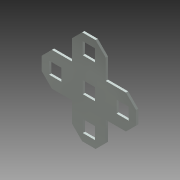
# Autodesk Inventor part: 276-1110
Saved by Autodesk Inventor 2013 (Build 170138000, 138)
## iProperties
Category: Structure
Company: Autodesk Inc.
Created: 2012-04-11
Part Number: 276-1110
Document SubType Name: Modeling
Designer: Autodesk Inc.
Density: 7.85 g/cm^3
Material: Steel
Catalog Web Link: http://www.vexrobotics.com/276-1110.html
Vendor: VEX
Mass: 3.81207 g
Surface Area: 13.3961 cm^2
Volume: 0.485614 cm^3
Author: Autodesk Inc.
Autodesk Inventor part; units mm, degrees
ref_plane "YZ Plane" through (0, 0, 0) normal (1, 0, 0) x (0, 1, 0)
ref_plane "XZ Plane" through (0, 0, 0) normal (0, 1, 0) x (-1, 0, 0)
ref_plane "XY Plane" through (0, 0, 0) normal (0, 0, 1) x (1, 0, 0)
sketch "Sketch1" plane through (0, 0, 0) normal (0, 0, 1) x (1, 0, 0)
  line L0 (20.9262, 6.7683) -> (20.9262, 1.6883)
  line L1 (-14.6338, 1.6883) -> (-14.6338, 6.7683)
  line L2 (0.6062, 22.0083) -> (5.6862, 22.0083)
  line L3 (5.6862, -13.5517) -> (0.6062, -13.5517)
  line L4 (-3.2038, -9.7417) -> (-3.2038, -2.1217)
  line L5 (-3.2038, 10.5783) -> (-3.2038, 18.1983)
  line L6 (-10.8238, 10.5783) -> (-3.2038, 10.5783)
  line L7 (9.4962, 10.5783) -> (17.1162, 10.5783)
  line L8 (17.1162, -2.1217) -> (9.4962, -2.1217)
  line L9 (-3.2038, -2.1217) -> (-10.8238, -2.1217)
  line L10 (9.4962, 18.1983) -> (9.4962, 10.5783)
  line L11 (9.4962, -2.1217) -> (9.4962, -9.7417)
  line L12 (-3.2038, 18.1983) -> (0.6062, 22.0083)
  line L13 (5.6862, 22.0083) -> (9.4962, 18.1983)
  line L14 (17.1162, 10.5783) -> (20.9262, 6.7683)
  line L15 (20.9262, 1.6883) -> (17.1162, -2.1217)
  line L16 (9.4962, -9.7417) -> (5.6862, -13.5517)
  line L17 (-3.2038, -9.7417) -> (0.6062, -13.5517)
  line L18 (-14.6338, 1.6883) -> (-10.8238, -2.1217)
  line L19 (-14.6338, 6.7683) -> (-10.8238, 10.5783)
  line L20 (0.8602, 19.2143) -> (5.4322, 19.2143)
  line L21 (5.4322, 19.2143) -> (5.4322, 14.6423)
  line L22 (5.4322, 14.6423) -> (0.8602, 14.6423)
  line L23 (0.8602, 14.6423) -> (0.8602, 19.2143)
  line L24 (-11.8398, 6.5143) -> (-7.2678, 6.5143)
  line L25 (-7.2678, 6.5143) -> (-7.2678, 1.9423)
  line L26 (-7.2678, 1.9423) -> (-11.8398, 1.9423)
  line L27 (-11.8398, 1.9423) -> (-11.8398, 6.5143)
  line L28 (0.8602, -6.1857) -> (5.4322, -6.1857)
  line L29 (5.4322, -6.1857) -> (5.4322, -10.7577)
  line L30 (5.4322, -10.7577) -> (0.8602, -10.7577)
  line L31 (0.8602, -10.7577) -> (0.8602, -6.1857)
  line L32 (13.5602, 6.5143) -> (18.1322, 6.5143)
  line L33 (18.1322, 6.5143) -> (18.1322, 1.9423)
  line L34 (18.1322, 1.9423) -> (13.5602, 1.9423)
  line L35 (13.5602, 1.9423) -> (13.5602, 6.5143)
  line L36 (0.8602, 6.5143) -> (5.4322, 6.5143)
  line L37 (5.4322, 6.5143) -> (5.4322, 1.9423)
  line L38 (5.4322, 1.9423) -> (0.8602, 1.9423)
  line L39 (0.8602, 1.9423) -> (0.8602, 6.5143)
  point P0 (-14.6338, 10.5783)
  point P1 (20.9262, -2.1217)
  point P2 (20.9262, 10.5783)
  point P3 (-14.6338, -2.1217)
  point P4 (-3.2038, 22.0083)
  point P5 (9.4962, -13.5517)
  point P6 (9.4962, 22.0083)
  point P7 (-3.2038, -13.5517)
  dimension "d0" = 35.56
  dimension "d1" = 35.56
  dimension "d2" = 12.7
  dimension "d3" = 12.7
  dimension "d4" = 12.7
  dimension "d5" = 12.7
  dimension "d6" = 11.43
  dimension "d7" = 11.43
  dimension "d8" = 11.43
  dimension "d9" = 11.43
  dimension "d10" = 3.81
  dimension "d11" = 3.81
  dimension "d12" = 3.81
  dimension "d13" = 3.81
  dimension "d14" = 3.81
  dimension "d15" = 3.81
  dimension "d16" = 3.81
  dimension "d17" = 3.81
  dimension "d18" = 3.81
  dimension "d19" = 3.81
  dimension "d20" = 3.81
  dimension "d21" = 3.81
  dimension "d22" = 3.81
  dimension "d23" = 3.81
  dimension "d24" = 3.81
  dimension "d25" = 3.81
  dimension "d26" = 4.572
  dimension "d27" = 4.572
  dimension "d28" = 4.572
  dimension "d29" = 4.572
  dimension "d30" = 4.572
  dimension "d31" = 4.572
  dimension "d32" = 4.572
  dimension "d33" = 4.572
  dimension "d34" = 4.572
  dimension "d35" = 4.572
  dimension "d36" = 2.794
  dimension "d37" = 2.794
  dimension "d38" = 2.794
  dimension "d39" = 2.794
  dimension "d40" = 4.064
  dimension "d41" = 4.064
  dimension "d42" = 11.43
  constraints: 80 end point, 20 parallel, 16 point on line, 9 perpendicular, 8 horizontal, 4 collinear
  measures "d0" distance between parallel lines of L0 L1
  measures "d1" distance between parallel lines of L3 L2
  measures "d2" distance of point (-3.204, 22.008) point (9.496, 22.008)
  measures "d3" distance of point (-14.634, -2.122) point (-14.634, 10.578)
  measures "d4" distance of point (20.926, 10.578) point (20.926, -2.122)
  measures "d5" distance of point (9.496, -13.552) point (-3.204, -13.552)
  measures "d6" distance of L5.start point (-3.204, 22.008)
  measures "d7" distance of point (-3.204, -13.552) L4.end
  measures "d8" distance of L8.end point (9.496, -13.552)
  measures "d9" distance of point (-14.634, 10.578) L5.start
  measures "d10" distance of L5.end point (-3.204, 22.008)
  measures "d11" distance of L2.start point (-3.204, 22.008)
  measures "d12" distance of L2.end point (9.496, 22.008)
  measures "d13" distance of L10.start point (9.496, 22.008)
  measures "d14" distance of L7.end point (20.926, 10.578)
  measures "d15" distance of L0.start point (20.926, 10.578)
  measures "d16" distance of L0.end point (20.926, -2.122)
  measures "d17" distance of L8.start point (20.926, -2.122)
  measures "d18" distance of L11.end point (9.496, -13.552)
  measures "d19" distance of L3.start point (9.496, -13.552)
  measures "d20" distance of L4.start point (-3.204, -13.552)
  measures "d21" distance of L3.end point (-3.204, -13.552)
  measures "d22" distance of L1.start point (-14.634, -2.122)
  measures "d23" distance of L9.end point (-14.634, -2.122)
  measures "d24" distance of L1.end point (-14.634, 10.578)
  measures "d25" distance of L6.start point (-14.634, 10.578)
  measures "d26" distance of L21.end L22.end
  measures "d27" distance of L22.end L20.start
  measures "d28" distance of L24.end L25.end
  measures "d29" distance of L24.start L24.end
  measures "d30" distance of L36.start L36.end
  measures "d31" distance of L38.end L36.start
  measures "d32" distance of L34.end L32.start
  measures "d33" distance of L33.end L34.end
  measures "d34" distance of L28.start L28.end
  measures "d35" distance of L30.end L28.start
  measures "d36" distance between parallel lines of L1 L27
  measures "d37" distance between parallel lines of L2 L20
  measures "d38" distance between parallel lines of L3 L30
  measures "d39" distance between parallel lines of L0 L33
  measures "d40" distance between parallel lines of L7 L32
  measures "d41" distance between parallel lines of L11 L29
  measures "d42" distance between parallel lines of L4 L1
extrude "Extrusion1" add sketch "Sketch1" along normal blind 0.8382
sketch "Sketch2" plane through (0, 0, 0.8382) normal (0, 0, 1) x (1, 0, 0)
  line L0 (5.4322, 19.2143) -> (5.4322, 14.6423) projected
  line L1 (5.4322, 14.6423) -> (0.8602, 14.6423) projected
  line L2 (0.8602, 14.6423) -> (0.8602, 19.2143) projected
  line L3 (0.8602, 19.2143) -> (5.4322, 19.2143) projected
  circle A0 centre (3.1462, 16.9283) radius 2.286
  point P0 (0, 0)
  constraints: 4 tangent, 1 centre point
surface extrude "ExtrusionSrf1" sketch "Sketch2" against normal up to surface (0.8382 mm away) shown no curves A0
pattern_linear "Rectangular Pattern1" count 3 spacing 12.7 along (0, -1, 0) of "ExtrusionSrf1"
sketch "Sketch3" plane through (0, 0, 0.8382) normal (0, 0, 1) x (1, 0, 0)
  line L0 (-7.2678, 6.5143) -> (-7.2678, 1.9423) projected
  line L1 (-7.2678, 1.9423) -> (-11.8398, 1.9423) projected
  line L2 (-11.8398, 1.9423) -> (-11.8398, 6.5143) projected
  line L3 (-11.8398, 6.5143) -> (-7.2678, 6.5143) projected
  circle A0 centre (-9.5538, 4.2283) radius 2.286
  point P0 (0, 0)
  constraints: 4 tangent, 1 centre point
surface extrude "ExtrusionSrf4" sketch "Sketch3" against normal up to surface (0.8382 mm away) shown no curves A0
pattern_linear "Rectangular Pattern2" count 2 spacing 25.4 along (1, 0, 0) of "ExtrusionSrf4"
equation "\"d11\" = d10"
equation "\"d12\" = d10"
equation "\"d13\" = d12"
equation "\"d14\" = d10"
equation "\"d15\" = d14"
equation "\"d16\" = d10"
equation "\"d17\" = d16"
equation "\"d18\" = d10"
equation "\"d19\" = d18"
equation "\"d20\" = d10"
equation "\"d21\" = d20"
equation "\"d22\" = d10"
equation "\"d23\" = d22"
equation "\"d24\" = d10"
equation "\"d25\" = d24"
body "Solid1"
body "Srf1"
body "Srf2"
body "Srf3"
body "Srf4"
body "Srf5"
